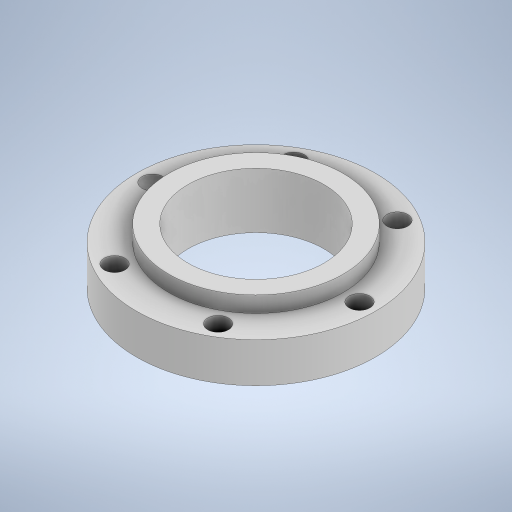
# Autodesk Inventor part: OsKrepl
Saved by Autodesk Inventor 2024 (Build 280153000, 153)
## iProperties
Created: 2023-08-20
Part Number: OsKrepl
Material: Generic
Document SubType Name: Modeling
Designer: KirikDK
Density: 1 g/cm^3
Appearance: Default
Author: KirikDK
Autodesk Inventor part; units mm, degrees
ref_plane "YZ Plane" through (0, 0, 0) normal (1, 0, 0) x (0, 1, 0)
ref_plane "XZ Plane" through (0, 0, 0) normal (0, 1, 0) x (-1, 0, 0)
ref_plane "XY Plane" through (0, 0, 0) normal (0, 0, 1) x (1, 0, 0)
sketch "Sketch1" plane through (0, 0, 0) normal (0, 1, 0) x (-1, 0, 0)
  arc A0 (11.4577, 20.6245) -> (5.4577, 24.5686) centre (0.4577, 10.4265) ccw
  circle A1 centre (0.4577, 10.4265) radius 15
  circle A2 centre (13.4577, 10.4265) radius 1.3
  circle A3 centre (6.9577, 21.6848) radius 1.3
  circle A4 centre (-6.0423, 21.6848) radius 1.3
  circle A5 centre (-12.5423, 10.4265) radius 1.3
  circle A6 centre (-6.0423, -0.8319) radius 1.3
  circle A7 centre (6.9577, -0.8319) radius 1.3
  circle A8 centre (0.4577, 10.4265) radius 8.5423
  point P0 (0, 0)
  point P1 (0.4577, 10.4265)
  dimension "d2" = 2.6
  dimension "d3" = 13
  dimension "d4" = 360
  constraints: 8 centre point, 2 coincident, 2 point on circle, 16 other
  measures "d2" diameter of A2
  measures "d3" distance of A2.centre point (0.458, 10.426)
extrude "Extrusion1" add sketch "Sketch1" along normal blind 5
sketch "Sketch2" plane through (-0.4577, 5, 10.4265) normal (0, 1, 0) x (1, 0, 0)
  circle A0 centre (0, 0) radius 10.95
  circle A1 centre (0, 0) radius 8.5423
  point P0 (0.4577, 10.4265)
  dimension "d7" = 21.9
  constraints: 2 centre point, 1 coincident
  measures "d7" diameter of A0
extrude "Extrusion2" add sketch "Sketch2" along normal blind 2
body "Solid1"
